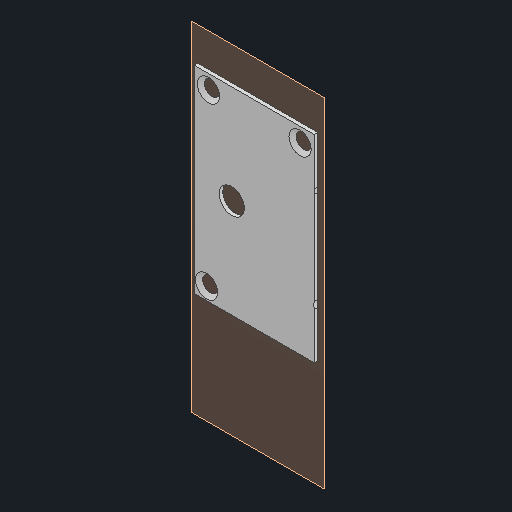
# Autodesk Inventor part: right_metal_gear_bracker
Saved by Autodesk Inventor 2023 (Build 270158000, 158)
## iProperties
Created: 2024-04-23
Part Number: right_metal_gear_bracker
Material: Generic
Document SubType Name: Modeling
Designer: szymo
Density: 1 g/cm^3
Appearance: Default
Author: szymo
Autodesk Inventor part; units mm, degrees
ref_plane "YZ Plane" through (0, 0, 0) normal (1, 0, 0) x (0, 1, 0)
ref_plane "XZ Plane" through (0, 0, 0) normal (0, 1, 0) x (-1, 0, 0)
ref_plane "XY Plane" through (0, 0, 0) normal (0, 0, 1) x (1, 0, 0)
ref_plane "Work Plane1" through (3, 4, -1) normal (0, 0, 1) x (0, -1, 0)
sketch "Sketch1" plane through (3, 4, -1) normal (0, 0, 1) x (0, -1, 0)
  line L0 (18.0177, 33.5) -> (5, 33.5)
  line L1 (5, 0) -> (5, 33.5)
  line L2 (5, 0) -> (89.75, 0)
  line L3 (89.75, 0) -> (89.75, 33.5)
  line L4 (5, 0) -> (60, 0)
  line L5 (5, -3) -> (5, 0)
  line L6 (4, -3) -> (60, -3)
  line L7 (60, 33.5) -> (60, 0)
  line L8 (60, -3) -> (60, 0)
  line L9 (60, 0) -> (183, 0)
  circle A0 centre (74.375, 17.375) radius 6.75
  line L10 (60, 0) -> (60, 33.5)
  circle A1 centre (32.5, 10.5) radius 5.5
  circle A2 centre (9, 4) radius 2.1
  circle A3 centre (9, 29.5) radius 2.1
  circle A4 centre (56.5, 3.5) radius 2.1
  spline S0 degree 2 poles (19.3669, 33.5) (18.6923, 33.3555) (18.0177, 33.5) knots 0 0 0 1 1 1 weights 1 1.02375 1
  line L11 (89.75, 33.5) -> (85.2105, 33.5)
  spline S1 degree 2 poles (85.2105, 33.5) (84.25, 33.2071) (83.2895, 33.5) knots 0 0 0 1 1 1 weights 1 1.05 1
  line L12 (83.2895, 33.5) -> (65.5855, 33.5)
  spline S2 degree 2 poles (65.5855, 33.5) (64.625, 33.2071) (63.6645, 33.5) knots 0 0 0 1 1 1 weights 1 1.05 1
  line L13 (63.6645, 33.5) -> (47.1605, 33.5)
  spline S3 degree 2 poles (47.1605, 33.5) (46.2, 33.2071) (45.2395, 33.5) knots 0 0 0 1 1 1 weights 1 1.05 1
  line L14 (45.2395, 33.5) -> (19.3669, 33.5)
  line L15 (183, 0) -> (183, 4.5)
  line L16 (183, 4.5) -> (137.8889, 33.5)
  line L17 (137.8889, 33.5) -> (60, 33.5)
  point P0 (52, 0)
  point P1 (64.076, 0)
  point P2 (87.674, 0)
  point P3 (63.25, 3.25)
  point P4 (60, 3.25)
  constraints: 2 end point, 1 perpendicular
extrude "Extrusion1" add sketch "Sketch1" along normal blind 1 contours S0 L14 S3 L13 L7 L2 L1 L0 | A1 | A2 | A3 | A4
sketch "Sketch2" plane through (3, 4, 0) normal (0, 0, 1) x (1, 0, 0)
  line L0 (12.5287, -34.71) -> (8.4496, -34.6899)
  arc A0 (8.4713, -30.29) -> (8.4496, -34.6899) centre (10.5, -32.5) ccw
  line L1 (8.4713, -30.29) -> (12.5504, -30.3101)
  arc A1 (12.5287, -34.71) -> (12.5504, -30.3101) centre (10.5, -32.5) ccw
  circle A2 centre (10.5, -32.5) radius 3
  circle A3 centre (10.5, -32.5) radius 3.5
  point P0 (-3, -4)
  dimension "d5" = 0.5
  constraints: 4 centre point, 4 end point, 4 point on circle, 1 coincident, 1 concentric, 10 other
  measures "d5" radial gap between concentric circles of A2 A3
extrude "Extrusion2" cut sketch "Sketch2" against normal up to next contours A2 L0 | L0 A0 L1 A1 | A2 L1 | A3
sketch "Sketch3" plane through (3, 4, 0) normal (0, 0, 1) x (1, 0, 0)
  circle A0 centre (10.5, -32.5) radius 3.5 projected
  line L0 (0, -5) -> (0, -60) projected
  line L1 (33.5, -18.0177) -> (33.5, -5) projected
  line L2 (33.5, -5) -> (0, -5) projected
  circle A1 centre (3.5, -56.5) radius 3.5
  circle A2 centre (4, -9) radius 4
  circle A3 centre (3.5, -56.5) radius 2.6
  circle A4 centre (4, -9) radius 2.6
  circle A5 centre (29.5, -9) radius 4
  circle A6 centre (29.5, -9) radius 2.6
  line L3 (33.5, -60) -> (33.5, -47.1605) projected
  line L4 (33.5, -45.2395) -> (33.5, -19.3669) projected
  line L5 (0, -60) -> (33.5, -60) projected
  point P0 (-3, -4)
  dimension "d8" = 7
  dimension "d17" = 8
  dimension "d18" = 5.2
  dimension "d19" = 5.2
  dimension "d20" = 4
  dimension "d21" = 4
  dimension "d22" = 8
  dimension "d23" = 5.2
  dimension "d24" = 4
  dimension "d25" = 4
  constraints: 6 centre point, 3 coincident, 2 vertical alignment, 1 tangent
  measures "d8" diameter of A1
  measures "d17" diameter of A2
  measures "d18" diameter of A3
  measures "d19" diameter of A4
  measures "d20" distance from line of L2 A2.centre
  measures "d21" distance from line of L0 A2.centre
  measures "d22" diameter of A5
  measures "d23" diameter of A6
  measures "d24" distance from line of L1 A5.centre
  measures "d25" distance from line of L2 A5.centre
hole "Hole1" at (6.5, -52.5, 0) at (7, -5, 0) at (32.5, -5, 0) direction (0, 0, -1) diameter 3.6 end through all countersink diameter 6.2 countersink angle 90 clearance for "Countersunk Flat Head Screw ISO 2009/7046" size "M3" standard "ISO"
body "Solid1"
